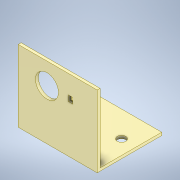
# Autodesk Inventor part: POT mount
Saved by Autodesk Inventor 2020.4 (Build 244396000, 396)
## iProperties
Created: 2022-04-16
Part Number: POT mount
Material: Nylon 6/6
Document SubType Name: Modeling
Designer: Gurkin
Density: 1.13 g/cm^3
Appearance: Nylon 6
Author: Gurkin
Autodesk Inventor part; units mm, degrees
ref_plane "YZ Plane" through (0, 0, 0) normal (1, 0, 0) x (0, 1, 0)
ref_plane "XZ Plane" through (0, 0, 0) normal (0, 1, 0) x (-1, 0, 0)
ref_plane "XY Plane" through (0, 0, 0) normal (0, 0, 1) x (1, 0, 0)
sketch "Sketch1" plane through (0, 0, 0) normal (0, 0, 1) x (1, 0, 0)
  line L0 (0, 0) -> (55, 0)
  line L1 (55, 0) -> (55, 50)
  line L2 (55, 50) -> (0, 50)
  line L3 (0, 50) -> (0, 0)
  dimension "d3" = 55
  dimension "d4" = 50
  constraints: 8 end point, 2 parallel, 1 horizontal, 1 perpendicular
  measures "d3" distance between parallel lines of L1 L3
  measures "d4" distance between parallel lines of L0 L2
extrude "Extrusion1" add sketch "Sketch1" along normal blind 2
sketch "Sketch2" plane through (0, 0, 2) normal (0, 0, 1) x (1, 0, 0)
  circle A0 centre (20, 35) radius 8
  line L0 (0, 0) -> (55, 0) projected
  line L1 (0, 50) -> (0, 0) projected
  line L2 (35, 37) -> (38, 37)
  line L3 (38, 37) -> (38, 33)
  line L4 (38, 33) -> (35, 33)
  line L5 (35, 33) -> (35, 37)
  dimension "d2" = 16
  dimension "d5" = 35
  dimension "d6" = 20
  dimension "d7" = 15
  dimension "d8" = 4
  dimension "d9" = 3
  dimension "d10" = 2
  constraints: 8 end point, 2 parallel, 1 centre point, 1 horizontal, 1 perpendicular
  measures "d2" diameter of A0
  measures "d5" distance from line of L0 A0.centre
  measures "d6" distance from line of L1 A0.centre
  measures "d7" distance from line of L5 A0.centre
  measures "d8" distance between parallel lines of L4 L2
  measures "d9" distance between parallel lines of L5 L3
  measures "d10" distance from line of A0.centre L4
extrude "Extrusion2" cut sketch "Sketch2" against normal through all
sketch "Sketch4" plane through (0, 0, 2) normal (0, 0, 1) x (1, 0, 0)
  line L0 (0, 2) -> (0, 0)
  line L1 (0, 0) -> (55, 0)
  line L2 (55, 0) -> (55, 2)
  line L3 (55, 2) -> (0, 2)
  line L4 (0, 2) -> (0, 0)
  dimension "d26" = 2
  dimension "d27" = 55
  constraints: 10 end point, 2 parallel, 1 horizontal, 1 perpendicular
  measures "d26" distance between parallel lines of L1 L3
  measures "d27" distance between parallel lines of L2 L0
extrude "Extrusion3" add sketch "Sketch4" against normal blind 45
sketch "Sketch6" plane through (0, 2, 0) normal (0, 1, 0) x (1, 0, 0)
  circle A0 centre (10, 25) radius 3
  circle A1 centre (45, 25) radius 3
  line L0 (0, 0) -> (0, 43) projected
  line L1 (55, 0) -> (55, 43) projected
  line L2 (0, 43) -> (55, 43) projected
  dimension "d28" = 6
  dimension "d29" = 6
  dimension "d30" = 10
  dimension "d31" = 10
  dimension "d32" = 18
  dimension "d33" = 18
  constraints: 2 centre point
  measures "d28" diameter of A0
  measures "d29" diameter of A1
  measures "d30" distance from line of L0 A0.centre
  measures "d31" distance from line of L1 A1.centre
  measures "d32" distance from line of L2 A0.centre
  measures "d33" distance from line of L2 A1.centre
extrude "Extrusion5" cut sketch "Sketch6" against normal through all
body "Solid1"
